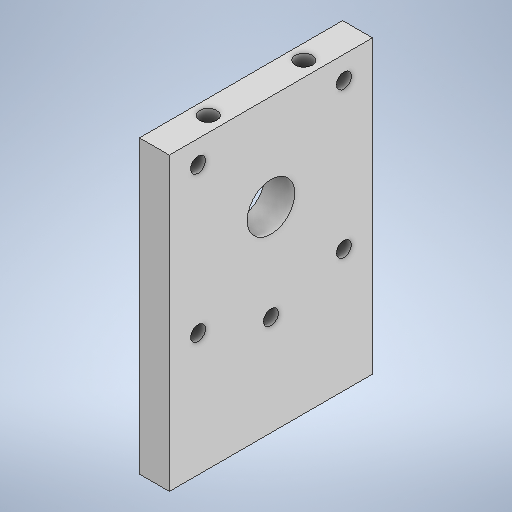
# Autodesk Inventor part: Bracket(left)
Saved by Autodesk Inventor 2025.1 (Build 291241020, 241B)
## iProperties
Created: 2025-01-21
Part Number: Bracket(left)
Material: Generic
Document SubType Name: Modeling
Designer: Sven
Density: 1 g/cm^3
Appearance: Default
Author: Sven
Autodesk Inventor part; units mm, degrees
ref_plane "YZ Plane" through (0, 0, 0) normal (1, 0, 0) x (0, 1, 0)
ref_plane "XZ Plane" through (0, 0, 0) normal (0, 1, 0) x (-1, 0, 0)
ref_plane "XY Plane" through (0, 0, 0) normal (0, 0, 1) x (1, 0, 0)
sketch "Sketch1" plane through (0, 0, 0) normal (0, 0, 1) x (1, 0, 0)
  line L0 (-139.7, 31.75) -> (139.7, 31.75)
  line L1 (139.7, 31.75) -> (139.7, -31.75)
  line L2 (139.7, -31.75) -> (-139.7, -31.75)
  line L3 (-139.7, -31.75) -> (-139.7, 31.75)
  point P0 (0, 0)
  point P1 (0, 31.75)
  point P2 (139.7, 0)
  dimension "d0" = 279.4
  dimension "d1" = 63.5
  constraints: 8 end point, 2 midpoint, 2 parallel, 1 horizontal, 1 horizontal alignment, 1 perpendicular, 1 vertical alignment
  measures "d0" distance of L0.start L0.end
  measures "d1" distance of L0.end L1.end
extrude "Extrusion1" add sketch "Sketch1" along normal blind 43.18
sketch "Sketch2" plane through (0, 0, 43.18) normal (0, 0, 1) x (1, 0, 0)
  line L0 (-139.7, -31.75) -> (139.7, -31.75) projected
  line L1 (-138.1125, 30.1625) -> (138.1125, 30.1625)
  line L2 (138.1125, 30.1625) -> (138.1125, -31.75)
  line L3 (138.1125, -31.75) -> (-138.1125, -31.75)
  line L4 (-138.1125, -31.75) -> (-138.1125, 30.1625)
  line L5 (139.7, -31.75) -> (139.7, 31.75) projected
  line L6 (139.7, 31.75) -> (-139.7, 31.75) projected
  line L7 (-139.7, 31.75) -> (-139.7, -31.75) projected
  point P0 (0, 0)
  point P1 (-138.1125, -31.75)
  dimension "d4" = 1.5875
  dimension "d5" = 1.5875
  dimension "d6" = 1.5875
  constraints: 8 end point, 2 parallel, 1 horizontal, 1 perpendicular, 1 point on line
  measures "d4" distance between parallel lines of L5 L2
  measures "d5" distance between parallel lines of L6 L1
  measures "d6" distance between parallel lines of L7 L4
extrude "Extrusion2" cut sketch "Sketch2" against normal up to surface (43.18 mm away) contours L4 L1 L2 L0
sketch "Sketch3" plane through (-138.1125, -31.75, 43.18) normal (1, 0, 0) x (0, 0, -1)
  circle A0 centre (21.59, 41.5925) radius 5.05
  line L0 (0, 61.9125) -> (43.18, 61.9125) projected
  circle A1 centre (21.59, 21.2725) radius 1.5875
  line L1 (43.18, 63.5) -> (0, 63.5) projected
  point P0 (43.18, 31.75)
  point P1 (21.59, 63.5)
  dimension "d9" = 10.1
  dimension "d10" = 20.32
  dimension "d13" = 3.175
  dimension "d15" = 20.32
  constraints: 2 centre point, 2 vertical alignment, 1 midpoint
  measures "d9" diameter of A0
  measures "d10" distance from line of L0 A0.centre
  measures "d13" diameter of A1
  measures "d15" distance of A1.centre A0.centre
extrude "Extrusion3" cut sketch "Sketch3" along normal through all both and the other way through all
sketch "Sketch4" plane through (139.7, -31.75, 0) normal (1, 0, 0) x (0, 0, -1)
  circle A0 centre (-10.16, 26.3525) radius 2.3813
  line L0 (0, 63.5) -> (-43.18, 63.5) construction
  line L1 (-21.59, 63.5) -> (-21.59, -3.1611) construction
  line L2 (0, 0) -> (0, 63.5) projected
  circle A1 centre (-21.59, 41.5925) radius 5.05 projected
  circle A2 centre (-33.02, 26.3525) radius 2.3813
  point P0 (0, 31.75)
  dimension "d16" = 10.16
  dimension "d17" = 15.24
  dimension "d18" = 4.7625
  constraints: 2 centre point, 2 end point, 1 midpoint, 1 symmetric about line, 1 vertical, 1 other
  measures "d16" distance from line of L2 A0.centre
  measures "d17" vertical distance of A1.centre A0.centre
  measures "d18" diameter of A0
extrude "Extrusion4" cut sketch "Sketch4" against normal up to surface (1.5875 mm away) contours A0 | A2
sketch "Sketch5" plane through (-139.7, -31.75, 0) normal (-1, 0, 0) x (0, 0, 1)
  circle A0 centre (21.59, 41.5925) radius 5.05 construction
  line L0 (21.59, 41.5925) -> (21.59, 66.4825) construction
  line L1 (21.59, 41.5925) -> (51.2225, 41.5925) construction
  circle A1 centre (37.09, 57.0925) radius 1.5875
  circle A2 centre (6.09, 57.0925) radius 1.5875
  circle A3 centre (37.09, 26.0925) radius 1.5875
  circle A4 centre (6.09, 26.0925) radius 1.5875
  point P0 (0, 31.75)
  dimension "d21" = 3.175
  dimension "d22" = 15.5
  dimension "d23" = 15.5
  constraints: 4 centre point, 4 end point, 3 symmetric about line, 1 horizontal, 1 vertical, 3 other
  measures "d21" diameter of A1
  measures "d22" distance from line of L1 A1.centre
  measures "d23" distance from line of L0 A1.centre
extrude "Extrusion5" cut sketch "Sketch5" against normal up to surface (1.5875 mm away)
sketch "Sketch6" plane through (0, 0, 43.18) normal (0, 0, 1) x (1, 0, 0)
  line L0 (-138.1125, 30.1625) -> (138.1125, 30.1625) projected
  line L1 (-138.1125, 30.1625) -> (155.4569, 30.1625)
  line L2 (155.4569, 30.1625) -> (155.4569, 53.3555)
  line L3 (155.4569, 53.3555) -> (-138.1125, 53.3555)
  line L4 (-138.1125, 53.3555) -> (-138.1125, 30.1625)
  line L5 (155.4569, 53.3555) -> (81.9347, 53.3555)
  line L6 (81.9347, 53.3555) -> (81.9347, -39.2964)
  line L7 (81.9347, -39.2964) -> (155.4569, -39.2964)
  line L8 (155.4569, -39.2964) -> (155.4569, 53.3555)
  line L9 (-138.1125, 30.1625) -> (-141.389, 30.1625)
  line L10 (-141.389, 30.1625) -> (-141.389, 34.0033)
  line L11 (-141.389, 34.0033) -> (-138.1125, 34.0033)
  line L12 (-138.1125, 34.0033) -> (-138.1125, 30.1625)
  point P0 (0, 0)
  point P1 (81.9347, 30.1625)
  constraints: 24 end point, 6 parallel, 3 horizontal, 3 perpendicular
extrude "Extrusion6" cut sketch "Sketch6" against normal through all
sketch "Sketch7" plane through (-139.7, -31.75, 0) normal (-1, 0, 0) x (0, 0, 1)
  line L0 (43.18, 61.9125) -> (0, 61.9125) projected
  line L1 (0, 61.9125) -> (0, 0) projected
  line L2 (0, 0) -> (43.18, 0) projected
  line L3 (43.18, 61.9125) -> (43.18, 0) projected
  circle A0 centre (37.09, 26.0925) radius 1.5875 projected
  circle A1 centre (6.09, 57.0925) radius 1.5875 projected
  circle A2 centre (6.09, 26.0925) radius 1.5875 projected
  circle A3 centre (37.09, 57.0925) radius 1.5875 projected
  circle A4 centre (21.59, 41.5925) radius 5.05 projected
  circle A5 centre (21.59, 21.2725) radius 1.5875 projected
  point P0 (0, 31.75)
extrude "Extrusion7" add sketch "Sketch7" against normal blind 6.35
sketch "Sketch8" plane through (-139.7, 30.1625, 43.18) normal (0, 1, 0) x (1, 0, 0)
  line L0 (0, 0) -> (6.35, 0) projected
  line L1 (3.175, 0) -> (3.175, 11.43)
  line L2 (0, 43.18) -> (6.35, 43.18) projected
  line L3 (3.175, 43.18) -> (3.175, 31.75)
  point P0 (139.7, 43.18)
  dimension "d30" = 11.43
  dimension "d31" = 11.43
  constraints: 4 end point, 2 coincident, 2 midpoint, 2 vertical
  measures "d30" distance of L1.start L1.end
  measures "d31" distance of L3.start L3.end
hole "Hole1" at (-136.525, 30.1625, 31.75) at (-136.525, 30.1625, 11.43) direction (0, -1, 0) diameter 3.6576 depth 22.479 tip angle 118 clearance for "Hex Machine Screw" size "#6" standard "Ansi Unified Screw Threads"
body "Solid1"
